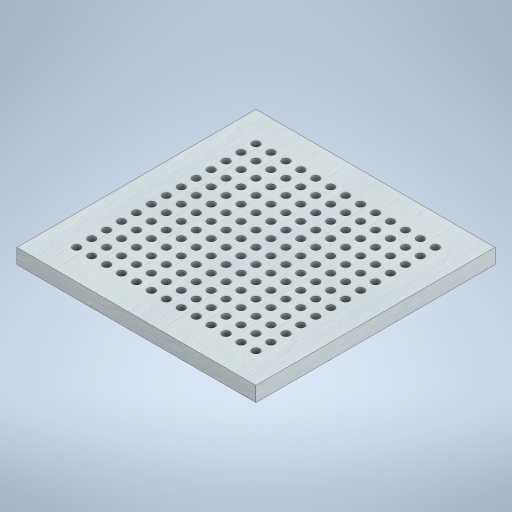
# Autodesk Inventor part: Box Lid
Saved by Autodesk Inventor 2023.1 (Build 271208000, 208)
## iProperties
Created: 2022-10-10
Part Number: Box Lid
Material: Wood (Oak)
Document SubType Name: Modeling
Designer: hudso
Density: 0.76 g/cm^3
Appearance: Wood - Painted White
Author: hudso
Autodesk Inventor part; units mm, degrees
ref_plane "YZ Plane" through (0, 0, 0) normal (1, 0, 0) x (0, 1, 0)
ref_plane "XZ Plane" through (0, 0, 0) normal (0, 1, 0) x (-1, 0, 0)
ref_plane "XY Plane" through (0, 0, 0) normal (0, 0, 1) x (1, 0, 0)
sketch "Sketch1" plane through (0, 0, 0) normal (0, 1, 0) x (-1, 0, 0)
  line L0 (-105.5896, 100.8203) -> (97.6104, 100.8203)
  line L1 (97.6104, 100.8203) -> (97.6104, -102.3797)
  line L2 (97.6104, -102.3797) -> (-105.5896, -102.3797)
  line L3 (-105.5896, -102.3797) -> (-105.5896, 100.8203)
  point P0 (0, 0)
  dimension "d0" = 203.2
  dimension "d1" = 203.2
  constraints: 8 end point, 2 parallel, 1 horizontal, 1 perpendicular
  measures "d0" distance of L1.end L2.end
  measures "d1" distance of L0.end L1.end
extrude "Extrusion1" add sketch "Sketch1" along normal blind 12.7
sketch "Sketch2" plane through (0, 12.7, 0) normal (0, 1, 0) x (1, 0, 0)
  point P0 (0, 0)
sketch "Sketch3" plane through (0, 12.7, 0) normal (0, 1, 0) x (1, 0, 0)
  line L0 (-84.9104, -88.1203) -> (92.8896, -88.1203)
  line L1 (92.8896, -88.1203) -> (92.8896, 89.6797)
  line L2 (92.8896, 89.6797) -> (-84.9104, 89.6797)
  line L3 (-84.9104, 89.6797) -> (-84.9104, -88.1203)
  line L4 (105.5896, 102.3797) -> (-97.6104, 102.3797) projected
  line L5 (-97.6104, 102.3797) -> (-97.6104, -100.8203) projected
  line L6 (-97.6104, -100.8203) -> (105.5896, -100.8203) projected
  line L7 (105.5896, -100.8203) -> (105.5896, 102.3797) projected
  circle A0 centre (-72.2104, 76.9797) radius 3.175
  line L8 (-72.2104, 76.9797) -> (-72.2104, -75.4203)
  line L9 (-72.2104, 76.9797) -> (80.1896, 76.9797)
  circle A1 centre (-72.2104, 64.2797) radius 3.175
  circle A2 centre (-72.2104, 51.5797) radius 3.175
  circle A3 centre (-72.2104, 38.8797) radius 3.175
  circle A4 centre (-72.2104, 26.1797) radius 3.175
  circle A5 centre (-72.2104, 13.4797) radius 3.175
  circle A6 centre (-72.2104, 0.7797) radius 3.175
  circle A7 centre (-72.2104, -11.9203) radius 3.175
  circle A8 centre (-72.2104, -24.6203) radius 3.175
  circle A9 centre (-72.2104, -37.3203) radius 3.175
  circle A10 centre (-72.2104, -50.0203) radius 3.175
  circle A11 centre (-72.2104, -62.7203) radius 3.175
  circle A12 centre (-72.2104, -75.4203) radius 3.175
  circle A13 centre (-59.5104, 76.9797) radius 3.175
  circle A14 centre (-59.5104, 64.2797) radius 3.175
  circle A15 centre (-59.5104, 51.5797) radius 3.175
  circle A16 centre (-59.5104, 38.8797) radius 3.175
  circle A17 centre (-59.5104, 26.1797) radius 3.175
  circle A18 centre (-59.5104, 13.4797) radius 3.175
  circle A19 centre (-59.5104, 0.7797) radius 3.175
  circle A20 centre (-59.5104, -11.9203) radius 3.175
  circle A21 centre (-59.5104, -24.6203) radius 3.175
  circle A22 centre (-59.5104, -37.3203) radius 3.175
  circle A23 centre (-59.5104, -50.0203) radius 3.175
  circle A24 centre (-59.5104, -62.7203) radius 3.175
  circle A25 centre (-59.5104, -75.4203) radius 3.175
  circle A26 centre (-46.8104, 76.9797) radius 3.175
  circle A27 centre (-46.8104, 64.2797) radius 3.175
  circle A28 centre (-46.8104, 51.5797) radius 3.175
  circle A29 centre (-46.8104, 38.8797) radius 3.175
  circle A30 centre (-46.8104, 26.1797) radius 3.175
  circle A31 centre (-46.8104, 13.4797) radius 3.175
  circle A32 centre (-46.8104, 0.7797) radius 3.175
  circle A33 centre (-46.8104, -11.9203) radius 3.175
  circle A34 centre (-46.8104, -24.6203) radius 3.175
  circle A35 centre (-46.8104, -37.3203) radius 3.175
  circle A36 centre (-46.8104, -50.0203) radius 3.175
  circle A37 centre (-46.8104, -62.7203) radius 3.175
  circle A38 centre (-46.8104, -75.4203) radius 3.175
  circle A39 centre (-34.1104, 76.9797) radius 3.175
  circle A40 centre (-34.1104, 64.2797) radius 3.175
  circle A41 centre (-34.1104, 51.5797) radius 3.175
  circle A42 centre (-34.1104, 38.8797) radius 3.175
  circle A43 centre (-34.1104, 26.1797) radius 3.175
  circle A44 centre (-34.1104, 13.4797) radius 3.175
  circle A45 centre (-34.1104, 0.7797) radius 3.175
  circle A46 centre (-34.1104, -11.9203) radius 3.175
  circle A47 centre (-34.1104, -24.6203) radius 3.175
  circle A48 centre (-34.1104, -37.3203) radius 3.175
  circle A49 centre (-34.1104, -50.0203) radius 3.175
  circle A50 centre (-34.1104, -62.7203) radius 3.175
  circle A51 centre (-34.1104, -75.4203) radius 3.175
  circle A52 centre (-21.4104, 76.9797) radius 3.175
  circle A53 centre (-21.4104, 64.2797) radius 3.175
  circle A54 centre (-21.4104, 51.5797) radius 3.175
  circle A55 centre (-21.4104, 38.8797) radius 3.175
  circle A56 centre (-21.4104, 26.1797) radius 3.175
  circle A57 centre (-21.4104, 13.4797) radius 3.175
  circle A58 centre (-21.4104, 0.7797) radius 3.175
  circle A59 centre (-21.4104, -11.9203) radius 3.175
  circle A60 centre (-21.4104, -24.6203) radius 3.175
  circle A61 centre (-21.4104, -37.3203) radius 3.175
  circle A62 centre (-21.4104, -50.0203) radius 3.175
  circle A63 centre (-21.4104, -62.7203) radius 3.175
  circle A64 centre (-21.4104, -75.4203) radius 3.175
  circle A65 centre (-8.7104, 76.9797) radius 3.175
  circle A66 centre (-8.7104, 64.2797) radius 3.175
  circle A67 centre (-8.7104, 51.5797) radius 3.175
  circle A68 centre (-8.7104, 38.8797) radius 3.175
  circle A69 centre (-8.7104, 26.1797) radius 3.175
  circle A70 centre (-8.7104, 13.4797) radius 3.175
  circle A71 centre (-8.7104, 0.7797) radius 3.175
  circle A72 centre (-8.7104, -11.9203) radius 3.175
  circle A73 centre (-8.7104, -24.6203) radius 3.175
  circle A74 centre (-8.7104, -37.3203) radius 3.175
  circle A75 centre (-8.7104, -50.0203) radius 3.175
  circle A76 centre (-8.7104, -62.7203) radius 3.175
  circle A77 centre (-8.7104, -75.4203) radius 3.175
  circle A78 centre (3.9896, 76.9797) radius 3.175
  circle A79 centre (3.9896, 64.2797) radius 3.175
  circle A80 centre (3.9896, 51.5797) radius 3.175
  circle A81 centre (3.9896, 38.8797) radius 3.175
  circle A82 centre (3.9896, 26.1797) radius 3.175
  circle A83 centre (3.9896, 13.4797) radius 3.175
  circle A84 centre (3.9896, 0.7797) radius 3.175
  circle A85 centre (3.9896, -11.9203) radius 3.175
  circle A86 centre (3.9896, -24.6203) radius 3.175
  circle A87 centre (3.9896, -37.3203) radius 3.175
  circle A88 centre (3.9896, -50.0203) radius 3.175
  circle A89 centre (3.9896, -62.7203) radius 3.175
  circle A90 centre (3.9896, -75.4203) radius 3.175
  circle A91 centre (16.6896, 76.9797) radius 3.175
  circle A92 centre (16.6896, 64.2797) radius 3.175
  circle A93 centre (16.6896, 51.5797) radius 3.175
  circle A94 centre (16.6896, 38.8797) radius 3.175
  circle A95 centre (16.6896, 26.1797) radius 3.175
  circle A96 centre (16.6896, 13.4797) radius 3.175
  circle A97 centre (16.6896, 0.7797) radius 3.175
  circle A98 centre (16.6896, -11.9203) radius 3.175
  circle A99 centre (16.6896, -24.6203) radius 3.175
  circle A100 centre (16.6896, -37.3203) radius 3.175
  circle A101 centre (16.6896, -50.0203) radius 3.175
  circle A102 centre (16.6896, -62.7203) radius 3.175
  circle A103 centre (16.6896, -75.4203) radius 3.175
  circle A104 centre (29.3896, 76.9797) radius 3.175
  circle A105 centre (29.3896, 64.2797) radius 3.175
  circle A106 centre (29.3896, 51.5797) radius 3.175
  circle A107 centre (29.3896, 38.8797) radius 3.175
  circle A108 centre (29.3896, 26.1797) radius 3.175
  circle A109 centre (29.3896, 13.4797) radius 3.175
  circle A110 centre (29.3896, 0.7797) radius 3.175
  circle A111 centre (29.3896, -11.9203) radius 3.175
  circle A112 centre (29.3896, -24.6203) radius 3.175
  circle A113 centre (29.3896, -37.3203) radius 3.175
  circle A114 centre (29.3896, -50.0203) radius 3.175
  circle A115 centre (29.3896, -62.7203) radius 3.175
  circle A116 centre (29.3896, -75.4203) radius 3.175
  circle A117 centre (42.0896, 76.9797) radius 3.175
  circle A118 centre (42.0896, 64.2797) radius 3.175
  circle A119 centre (42.0896, 51.5797) radius 3.175
  circle A120 centre (42.0896, 38.8797) radius 3.175
  circle A121 centre (42.0896, 26.1797) radius 3.175
  circle A122 centre (42.0896, 13.4797) radius 3.175
  circle A123 centre (42.0896, 0.7797) radius 3.175
  circle A124 centre (42.0896, -11.9203) radius 3.175
  circle A125 centre (42.0896, -24.6203) radius 3.175
  circle A126 centre (42.0896, -37.3203) radius 3.175
  circle A127 centre (42.0896, -50.0203) radius 3.175
  circle A128 centre (42.0896, -62.7203) radius 3.175
  circle A129 centre (42.0896, -75.4203) radius 3.175
  circle A130 centre (54.7896, 76.9797) radius 3.175
  circle A131 centre (54.7896, 64.2797) radius 3.175
  circle A132 centre (54.7896, 51.5797) radius 3.175
  circle A133 centre (54.7896, 38.8797) radius 3.175
  circle A134 centre (54.7896, 26.1797) radius 3.175
  circle A135 centre (54.7896, 13.4797) radius 3.175
  circle A136 centre (54.7896, 0.7797) radius 3.175
  circle A137 centre (54.7896, -11.9203) radius 3.175
  circle A138 centre (54.7896, -24.6203) radius 3.175
  circle A139 centre (54.7896, -37.3203) radius 3.175
  circle A140 centre (54.7896, -50.0203) radius 3.175
  circle A141 centre (54.7896, -62.7203) radius 3.175
  circle A142 centre (54.7896, -75.4203) radius 3.175
  circle A143 centre (67.4896, 76.9797) radius 3.175
  circle A144 centre (67.4896, 64.2797) radius 3.175
  circle A145 centre (67.4896, 51.5797) radius 3.175
  circle A146 centre (67.4896, 38.8797) radius 3.175
  circle A147 centre (67.4896, 26.1797) radius 3.175
  circle A148 centre (67.4896, 13.4797) radius 3.175
  circle A149 centre (67.4896, 0.7797) radius 3.175
  circle A150 centre (67.4896, -11.9203) radius 3.175
  circle A151 centre (67.4896, -24.6203) radius 3.175
  circle A152 centre (67.4896, -37.3203) radius 3.175
  circle A153 centre (67.4896, -50.0203) radius 3.175
  circle A154 centre (67.4896, -62.7203) radius 3.175
  circle A155 centre (67.4896, -75.4203) radius 3.175
  circle A156 centre (80.1896, 76.9797) radius 3.175
  circle A157 centre (80.1896, 64.2797) radius 3.175
  circle A158 centre (80.1896, 51.5797) radius 3.175
  circle A159 centre (80.1896, 38.8797) radius 3.175
  circle A160 centre (80.1896, 26.1797) radius 3.175
  circle A161 centre (80.1896, 13.4797) radius 3.175
  circle A162 centre (80.1896, 0.7797) radius 3.175
  circle A163 centre (80.1896, -11.9203) radius 3.175
  circle A164 centre (80.1896, -24.6203) radius 3.175
  circle A165 centre (80.1896, -37.3203) radius 3.175
  circle A166 centre (80.1896, -50.0203) radius 3.175
  circle A167 centre (80.1896, -62.7203) radius 3.175
  circle A168 centre (80.1896, -75.4203) radius 3.175
  point P0 (0, 0)
  dimension "d4" = 177.8
  dimension "d5" = 177.8
  dimension "d12" = 6.35
  dimension "d13" = 12.7
  dimension "d14" = 12.7
  dimension "d15" = 12.7
  dimension "d16" = 12.7
  dimension "d17" = 25.4
  dimension "d18" = 25.4
  dimension "d19" = 152.4
  dimension "d20" = 152.4
  dimension "d23" = 12.7
  dimension "d26" = 12.7
  constraints: 169 centre point, 12 end point, 3 horizontal, 2 parallel, 2 vertical, 1 perpendicular, 336 other
  measures "d4" distance of L2.end L1.end
  measures "d5" distance of L1.end L0.end
  measures "d12" diameter of A0
  measures "d13" distance between parallel lines of L5 L3
  measures "d14" distance between parallel lines of L4 L2
  measures "d15" distance between parallel lines of L6 L0
  measures "d16" distance between parallel lines of L7 L1
  measures "d17" distance from line of L5 L8.start
  measures "d18" distance from line of L4 L8.start
  measures "d19" distance of L8.start L8.end
  measures "d20" distance of L8.start L9.end
  measures "d23" distance of L8.start A1.centre
  measures "d26" distance of L8.start A13.centre
extrude "Extrusion2" cut sketch "Sketch3" against normal blind 12.7 contours L9 L8 A0 | A0 L8 L9
pattern_linear "Rectangular Pattern1" count 13 spacing 12.7 along (0, 0, 1) count 13 spacing 12.7 along (1, 0, 0) of "Extrusion2"
body "Solid1"
